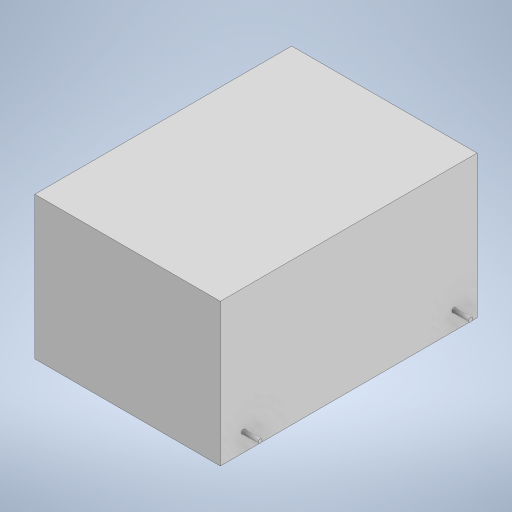
# Autodesk Inventor part: Frame
Saved by Autodesk Inventor 2023 (Build 270158000, 158)
## iProperties
Created: 2022-09-21
Part Number: Frame
Material: Generic
Document SubType Name: Modeling
Designer: PC
Density: 1 g/cm^3
Appearance: Default
Author: PC
Autodesk Inventor part; units mm, degrees
ref_plane "YZ Plane" through (0, 0, 0) normal (1, 0, 0) x (0, 1, 0)
ref_plane "XZ Plane" through (0, 0, 0) normal (0, 1, 0) x (-1, 0, 0)
ref_plane "XY Plane" through (0, 0, 0) normal (0, 0, 1) x (1, 0, 0)
sketch "Sketch1" plane through (0, 0, 0) normal (0, 0, 1) x (1, 0, 0)
  line L0 (0, 0) -> (660.4, 0)
  line L1 (660.4, 0) -> (660.4, 508)
  line L2 (660.4, 508) -> (0, 508)
  line L3 (0, 508) -> (0, 0)
  dimension "d0" = 660.4
  dimension "d1" = 508
  constraints: 8 end point, 2 parallel, 1 horizontal, 1 perpendicular
  measures "d0" distance of L2.end L1.end
  measures "d1" distance of L1.end L0.end
extrude "Extrusion1" add sketch "Sketch1" along normal blind 914.4
sketch "Sketch2" plane through (660.4, 0, 0) normal (1, 0, 0) x (0, 0, -1)
  circle A0 centre (-832.0024, 64.77) radius 7.3279
  line L0 (-914.4, 0) -> (-914.4, 508) projected
  line L1 (0, 0) -> (-914.4, 0) projected
  line L2 (0, 0) -> (-914.4, 0) projected
  line L3 (-457.2, 0) -> (-457.2, 118.7957)
  circle A1 centre (-82.3976, 64.77) radius 7.3279
  dimension "d4" = 14.6558
  dimension "d5" = 82.3976
  dimension "d6" = 64.77
  constraints: 2 centre point, 2 end point, 1 midpoint, 1 symmetric about line, 1 vertical, 1 other
  measures "d4" diameter of A0
  measures "d5" distance from line of L0 A0.centre
  measures "d6" distance from line of L1 A0.centre
extrude "Extrusion2" add sketch "Sketch2" along normal blind 59.0804
sketch "Sketch3" plane through (0, 0, 0) normal (-1, 0, 0) x (0, 0, 1)
  line L0 (0, 508) -> (0, 0) projected
  line L1 (0, 0) -> (914.4, 0) projected
  line L2 (914.4, 508) -> (914.4, 0) projected
  line L3 (0, 508) -> (914.4, 508) projected
  circle A0 centre (832.0024, 64.77) radius 7.3279 projected
  circle A1 centre (82.3976, 64.77) radius 7.3279 projected
extrude "Extrusion3" add sketch "Sketch3" along normal blind 59.0804 contours A0 | A1
body "Solid1"
